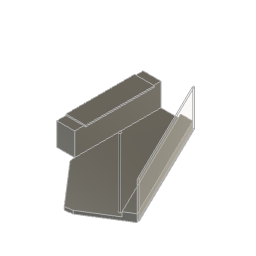
_Balkon.eec0943c-bb06-4ea9-9c15-2b337d19faf3 (Autodesk Fusion 360 design; units mm, degrees)
Autodesk Fusion 360 part; units mm, degrees
sketch "Sketch1" plane through (0, 0, 0) normal (0, 0, 1) x (1, 0, 0)
  line L0 (-10.0597, 280.8126) -> (89.9403, 280.8126)
  circle A0 centre (207.7788, -64.5249) radius 4.3
  line L1 (-8.4086, -5.102) -> (-10.0597, 10.8126)
  line L2 (-10.0597, 10.8126) -> (-10.0597, 280.8126)
  line L3 (89.9403, 280.8126) -> (254.3258, -57.3492)
  line L4 (254.3258, -57.3492) -> (130.5458, -134.3746)
  line L5 (130.5458, -134.3746) -> (106.5458, -138.3742)
  line L6 (106.5458, -138.3742) -> (-8.4086, -5.102)
  line L7 (51.58, 280.8126) -> (224.8744, -75.6761)
  dimension "d1" = 16
  dimension "d2" = 270
  dimension "d4" = 100
  dimension "d5" = 376
  dimension "d6" = 176
  dimension "d7" = 24
  dimension "d8" = 145.7889
  dimension "d11" = 34.5
  dimension "d26" = 8.6
  dimension "d27" = 18.5
  dimension "d28" = 45
  constraint coincident L1.start L6.end
  constraint vertical L2
  constraint coincident L0 L7.start
  constraint coincident L4 L7.end
  constraint parallel L3 L7
  constraint horizontal L0
  measures "d1" distance of L1.start L1.end
  measures "d2" vertical distance of L0.start L1.end
  measures "d4" distance of L0.start L0.end
  measures "d5" distance of L0.end L3.end
  measures "d6" distance of L5.end L1.start
  measures "d7" horizontal distance of L4.end L5.end
  measures "d8" distance of L3.end L4.end
  measures "d11" distance of L3 L7
  measures "d26" diameter of A0
  measures "d27" distance of A0.centre L4
  measures "d28" distance of A0.centre L3
extrude "Extrude1" add sketch "Sketch1" along normal blind 10 makes body 1
sketch "Sketch2" plane through (0, 0, 10) normal (0, 0, 1) x (-1, 0, 0)
  circle A0 centre (-207.7788, 64.5249) radius 4.3
  line L0 (-106.5458, 138.3742) -> (-130.5458, 134.3746)
  line L1 (-130.5458, 134.3746) -> (-254.3258, 57.3492)
  line L2 (-254.3258, 57.3492) -> (-89.9403, -280.8126)
  line L3 (-89.9403, -280.8126) -> (10.0597, -280.8126)
  line L4 (10.0597, -280.8126) -> (10.0597, -10.8126)
  line L5 (10.0597, -10.8126) -> (8.4086, 5.102)
  line L6 (8.4086, 5.102) -> (-106.5458, 138.3742)
  line L7 (-224.8744, 75.6761) -> (-51.58, -280.8126)
  line L8 (-89.9403, -280.8126) -> (-254.3258, 57.3492)
  line L9 (10.0597, -280.8126) -> (-89.9403, -280.8126)
  line L10 (-254.3258, 57.3492) -> (-130.5458, 134.3746)
  dimension "d12" = 34.5
  constraint coincident L1 L7.start
  constraint parallel L7 L8
  constraint coincident L7.end L9
  measures "d12" distance of L7 L8
extrude "Extrude2" add sketch "Sketch2" along normal blind 14 contours L1 L2 L3 L7 L8 L9 L10 bodies 1
sketch "Sketch3" plane through (0, 0, 10) normal (0, 0, 1) x (-1, 0, 0)
  line L0 (-224.8744, 75.6761) -> (-51.58, -280.8126)
  line L1 (-51.58, -280.8126) -> (10.0597, -280.8126)
  line L2 (10.0597, -280.8126) -> (10.0597, -10.8126)
  line L3 (10.0597, -10.8126) -> (8.4086, 5.102)
  line L4 (8.4086, 5.102) -> (-106.5458, 138.3742)
  line L5 (-106.5458, 138.3742) -> (-130.5458, 134.3746)
  line L6 (-130.5458, 134.3746) -> (-224.8744, 75.6761)
  circle A0 centre (-207.7788, 64.5249) radius 4.3
  line L7 (10.0597, -280.8126) -> (65.6684, -280.8126)
  line L8 (65.6684, -280.8126) -> (65.6684, -10.8126)
  line L9 (65.6684, -10.8126) -> (10.0597, -10.8126)
  constraint coincident L1.end L2.start
  constraint perpendicular L2 L7
  constraint perpendicular L7 L8
  constraint coincident L2.end L3.start
  constraint horizontal L9
extrude "Extrude3" add sketch "Sketch3" along normal blind 72.2 separate body contours L2 L7 L8 L9 makes body 2
sketch "Sketch4" plane through (0, 0, 82.2) normal (0, 0, 1) x (-1, 0, 0)
  line L0 (10.0597, -280.8126) -> (65.6684, -280.8126)
  line L1 (65.6684, -280.8126) -> (65.6684, -10.8126)
  line L2 (65.6684, -10.8126) -> (10.0597, -10.8126)
  line L3 (10.0597, -10.8126) -> (10.0597, -280.8126)
  line L4 (65.6684, -39.3126) -> (4.0597, -39.3126)
  line L5 (4.0597, -39.3126) -> (4.0597, -254.3126)
  line L6 (4.0597, -254.3126) -> (65.6684, -254.3126)
  line L7 (65.6684, -254.3126) -> (65.6684, -39.3126)
  line L8 (10.0597, -10.8126) -> (10.0597, -280.8126)
  dimension "d17" = 28.5
  dimension "d18" = 26.5
  dimension "d19" = 6
  constraint horizontal L4
  constraint vertical L5
  constraint horizontal L6
  constraint vertical L7
  constraint coincident L1 L4.start
  measures "d17" distance of L2 L4
  measures "d18" distance of L0 L6
  measures "d19" distance of L5 L8
extrude "Extrude4" add sketch "Sketch4" along normal blind 4 contours L3 L4 L5 L6 L8 | L1 L3 L4 L6 L7 L8 bodies 2
sketch "Sketch5" plane through (0, 0, 24) normal (0, 0, 1) x (-1, 0, 0)
  line L0 (-254.3258, 57.3492) -> (-89.9403, -280.8126)
  line L1 (-89.9403, -280.8126) -> (-51.58, -280.8126)
  line L2 (-51.58, -280.8126) -> (-224.8744, 75.6761)
  line L3 (-224.8744, 75.6761) -> (-254.3258, 57.3492)
  line L4 (-89.9403, -280.8126) -> (-93.5378, -282.5614)
  line L5 (-93.5378, -282.5614) -> (-257.0306, 53.764)
  line L6 (-257.0306, 53.764) -> (-254.3258, 57.3492)
  line L7 (-89.9403, -280.8126) -> (-254.3258, 57.3492)
  line L8 (-131.6451, 134.0722) -> (-133.5872, 137.1932)
  line L9 (-133.5872, 137.1932) -> (-259.6705, 58.7345)
  line L10 (-259.6705, 58.7345) -> (-257.0306, 53.764)
  line L11 (-254.3258, 57.3492) -> (-130.5458, 134.3746)
  dimension "d22" = 4
  dimension "d25" = 4
  constraint coincident L0.end L1.start
  constraint coincident L0.start L3.end
  constraint perpendicular L4 L5
  constraint parallel L5 L7
  constraint perpendicular L3 L8
  constraint perpendicular L8 L9
  measures "d22" distance of L0.end L4.end
  measures "d25" distance of L9 L11
extrude "Extrude5" add sketch "Sketch5" along normal blind 94.5 and the other way blind 20 separate body contours L0 L4 L5 L6 L7 makes body 3
extrude "Extrude6" add sketch "Sketch1" along normal blind 225 contours A0 bodies 1
sketch "Sketch6" plane through (0, 0, 10) normal (0, 0, 1) x (-1, 0, 0)
  line L0 (-224.8744, 75.6761) -> (-51.58, -280.8126)
  line L1 (-51.58, -280.8126) -> (10.0597, -280.8126)
  line L2 (10.0597, -280.8126) -> (10.0597, -10.8126)
  line L3 (10.0597, -10.8126) -> (8.4086, 5.102)
  line L4 (8.4086, 5.102) -> (-106.5458, 138.3742)
  line L5 (-106.5458, 138.3742) -> (-130.5458, 134.3746)
  line L6 (-130.5458, 134.3746) -> (-224.8744, 75.6761)
  circle A0 centre (-207.7788, 64.5249) radius 4.3
scale "Scale1" factor 10 about (224.8744, -75.6761, 24) bodies 1 2 3
